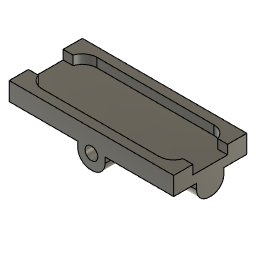
Leap_Motion_Mount (Autodesk Fusion 360 design; units mm, degrees)
Autodesk Fusion 360 part; units mm, degrees
sketch "Esquisse1" plane through (0, 0, 0) normal (0, 0, 1) x (1, 0, 0)
  line L0 (0, 0) -> (90, 0)
  line L1 (90, 0) -> (90, 40)
  line L2 (90, 40) -> (0, 40)
  line L3 (0, 40) -> (0, 0)
  line L4 (13, 35) -> (77, 35)
  line L5 (85, 27) -> (85, 13)
  line L6 (77, 5) -> (13, 5)
  line L7 (5, 13) -> (5, 27)
  arc A0 (13, 35) -> (5, 27) centre (13, 27) ccw
  arc A1 (85, 27) -> (77, 35) centre (77, 27) ccw
  arc A2 (77, 5) -> (85, 13) centre (77, 13) ccw
  arc A3 (5, 13) -> (13, 5) centre (13, 13) ccw
  line L8 (15, 0) -> (20, 0)
  line L9 (75, 0) -> (70, 0)
  line L10 (0, 29.5) -> (5.4007, 29.5)
  line L11 (0, 10.5) -> (5.4007, 10.5)
  line L12 (84.5993, 29.5) -> (90, 29.5)
  line L13 (84.5993, 10.5) -> (90, 10.5)
  dimension "d1" = 90
  dimension "d2" = 40
  dimension "d3" = 30
  dimension "d4" = 80
  dimension "d5" = 5
  dimension "d6" = 5
  dimension "d7" = 8
  dimension "d8" = 8
  dimension "d9" = 8
  dimension "d35" = 10.5
  dimension "d37" = 10.5
  dimension "d38" = 10.5
  dimension "d39" = 10.5
  constraint horizontal L0
  constraint vertical L1
  constraint horizontal L2
  constraint vertical L3
  constraint coincident L0.start L3.end
  constraint horizontal L4
  constraint vertical L5
  constraint horizontal L6
  constraint vertical L7
  constraint tangent L7 A0
  constraint tangent L4 A0
  constraint tangent L4 A1
  constraint tangent L5 A1
  constraint tangent L6 A2
  constraint tangent L5 A2
  constraint tangent L7 A3
  constraint tangent L6 A3
  constraint equal A2 A3
  constraint horizontal L8
  constraint coincident L0 L8.start
  constraint horizontal L9
  constraint coincident L0 L9.start
  constraint coincident L3 L10.start
  constraint coincident A0 L10.end
  constraint perpendicular L7 L10
  constraint coincident L3 L11.start
  constraint coincident A3 L11.end
  constraint perpendicular L3 L11
  constraint coincident A1 L12.start
  constraint coincident L1 L12.end
  constraint perpendicular L1 L12
  constraint coincident A2 L13.start
  constraint coincident L1 L13.end
  constraint perpendicular L1 L13
  measures "d1" distance of L0.start L0.end
  measures "d2" distance of L0 L2
  measures "d3" distance of L4 L6
  measures "d4" distance of L5 L7
  measures "d5" distance of L1 L5
  measures "d6" distance of L0 L6
  measures "d7" radius of A0
  measures "d8" radius of A1
  measures "d9" radius of A2
  measures "d35" distance of L2 L10
  measures "d37" distance of L0 L11
  measures "d38" distance of L2 L12
  measures "d39" distance of L0 L13
extrude "Extrusion18" cut sketch "Esquisse1" along normal blind 6
extrude "Extrusion19" cut sketch "Esquisse1" along normal blind 6
extrude "Extrusion33" add sketch "Esquisse1" along normal blind 5 separate body contours L3 L7 A0 A3 L10 L11 | L4 L5 L6 L7 A0 A1 A2 A3 | L1 L5 A1 A2 L12 L13
extrude "Extrusion34" add sketch "Esquisse1" along normal blind 10 contours L0 L1 L3 L6 A2 A3 L8 L9 L11 L13 | L1 L2 L3 L4 A0 A1 L10 L12
sketch "Esquisse16" plane through (0, 0, 0) normal (0, 0, 1) x (1, 0, 0)
  line L0 (0, 0) -> (90, 0)
  line L1 (90, 0) -> (90, 40)
  line L2 (90, 40) -> (0, 40)
  line L3 (0, 40) -> (0, 0)
  line L4 (52.5, 0) -> (37.5, 0)
  line L5 (37.5, 0) -> (37.5, 12.5)
  line L6 (52.5, 12.5) -> (52.5, 0)
  line L7 (0, 27.5) -> (15, 27.5)
  line L8 (15, 12.5) -> (0, 12.5)
  line L9 (0, 12.5) -> (0, 27.5)
  line L10 (15, 12.5) -> (37.5, 12.5)
  line L11 (37.5, 27.5) -> (37.5, 40)
  line L12 (52.5, 27.5) -> (52.5, 40)
  line L13 (52.5, 12.5) -> (90, 12.5)
  line L14 (15, 27.5) -> (37.5, 27.5)
  line L15 (52.5, 27.5) -> (90, 27.5)
  dimension "d215" = 37.5
  dimension "d216" = 15
  dimension "d218" = 15
  dimension "d220" = 12.5
  dimension "d221" = 40
  dimension "d222" = 90
  constraint horizontal L0
  constraint vertical L1
  constraint horizontal L2
  constraint vertical L3
  constraint coincident L0.start L3.end
  constraint horizontal L4
  constraint vertical L5
  constraint vertical L6
  constraint coincident L0 L4.start
  constraint horizontal L7
  constraint horizontal L8
  constraint vertical L9
  constraint coincident L3 L7.start
  constraint perpendicular L5 L10
  constraint coincident L2 L11.end
  constraint perpendicular L2 L11
  constraint coincident L2 L12.end
  constraint perpendicular L2 L12
  constraint coincident L1 L15.end
  constraint perpendicular L1 L14
  constraint coincident L1 L13.end
  constraint perpendicular L1 L13
  constraint coincident L12.start L14
  constraint collinear L14 L15
  measures "d215" distance of L3 L5
  measures "d216" distance of L5 L6
  measures "d218" distance of L7 L8
  measures "d220" distance of L0 L8
  measures "d221" distance of L0 L2
  measures "d222" distance of L0.start L0.end
extrude "Extrusion35" add sketch "Esquisse16" against normal blind 10 contours L0 L1 L2 L3 L4 L5 L6 L7 L8 L9 L10 L11 L12 L13 L14 L15 | L1 L2 L12 L15
sketch "Esquisse17" plane through (0, 0, 0) normal (0, -1, 0) x (1, 0, 0)
  line L0 (52.5, -10) -> (52.5, 0)
  line L1 (52.5, 0) -> (90, 0)
  line L2 (90, 0) -> (90, 10)
  line L3 (90, 10) -> (0, 10)
  line L4 (0, 10) -> (0, 0)
  line L5 (0, 0) -> (37.5, 0)
  line L6 (37.5, 0) -> (37.5, -10)
  circle A0 centre (45, -2) radius 3.5
  line L7 (37.5, -10) -> (52.5, -10)
  dimension "d229" = 7
  measures "d229" diameter of A0
extrude "Extrusion36" cut sketch "Esquisse17" against normal blind 13 contours A0
sketch "Esquisse18" plane through (0, 0, 0) normal (-1, 0, 0) x (0, -1, 0)
  line L0 (-12.5, -10) -> (-12.5, 0)
  line L1 (-12.5, 0) -> (0, 0)
  line L2 (0, 0) -> (0, 10)
  line L3 (0, 10) -> (-10.5, 10)
  line L4 (-10.5, 10) -> (-10.5, 5)
  line L5 (-10.5, 5) -> (-29.5, 5)
  line L6 (-29.5, 5) -> (-29.5, 10)
  line L7 (-29.5, 10) -> (-40, 10)
  line L8 (-40, 10) -> (-40, 0)
  line L9 (-40, 0) -> (-27.5, 0)
  line L10 (-27.5, 0) -> (-27.5, -10)
  circle A0 centre (-20, -2) radius 3.5
  line L11 (-27.5, -10) -> (-12.5, -10)
  dimension "d232" = 7
  measures "d232" diameter of A0
extrude "Extrusion37" cut sketch "Esquisse18" against normal blind 13 contours A0
extrude "Extrusion38" cut sketch "Esquisse16" against normal blind 10 contours L1 L2 L12 L15
fillet "Congé33" radius 7 8 edges at (18.75, 27.5, -10) (37.5, 33.75, -10) (52.5, 33.75, -10) (71.25, 27.5, -10) (71.25, 12.5, -10) (52.5, 6.25, -10) (37.5, 6.25, -10) (18.75, 12.5, -10)
equation "d5 = ( d1 - d4 ) / 2"
equation "d6 = ( d2 - d3 ) / 2"
equation "d7 = d9"
equation "d8 = d9"
equation "d35 = ( d2 - 19 mm ) / 2"
equation "d37 = d35"
equation "d38 = d35"
equation "d39 = d35"
equation "d215 = d222 / 2 - d216 / 2"
equation "d220 = d221 / 2 - d218 / 2"
named bodies: "Corps1"
